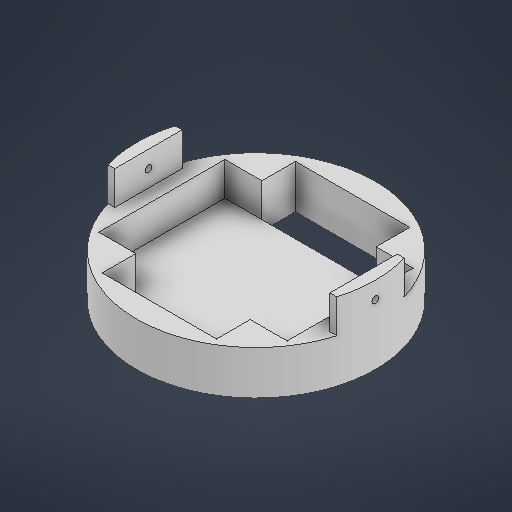
# Autodesk Inventor part: 007-002
Saved by Autodesk Inventor 2026 (Build 300175000, 175)
## iProperties
Created: 2026-04-20
Part Number: 007-002
Material: Ogólny
Document SubType Name: Modeling
Designer: Patryk Lombardo
Density: 1 g/cm^3
Appearance: Domyślna
Author: Patryk Lombardo
Autodesk Inventor part; units mm, degrees
ref_plane "YZ Plane" through (0, 0, 0) normal (1, 0, 0) x (0, 1, 0)
ref_plane "XZ Plane" through (0, 0, 0) normal (0, 1, 0) x (-1, 0, 0)
ref_plane "XY Plane" through (0, 0, 0) normal (0, 0, 1) x (1, 0, 0)
sketch "Szkic1" plane through (0, 0, 0) normal (0, 1, 0) x (-1, 0, 0)
  circle A0 centre (0, 0) radius 35.5
  line L0 (0, 18.75) -> (0, -18.75) construction
  line L1 (-28, 0) -> (28, 0) construction
  line L2 (-28, -18.75) -> (28, -18.75)
  line L3 (-28, 18.75) -> (-28, -18.75)
  line L4 (28, 18.75) -> (28, -18.75)
  line L5 (0, 18.75) -> (28, 18.75)
  line L6 (0, 18.75) -> (-28, 18.75)
  line L7 (0, 18.75) -> (0, 28.75) construction
  line L8 (17, 28.75) -> (-17, 28.75)
  line L9 (17, 28.75) -> (17, 18.75)
  line L10 (-17, 28.75) -> (-17, 18.75)
  line L11 (0, -18.75) -> (0, -28.75) construction
  line L12 (-17, -28.75) -> (17, -28.75)
  line L13 (17, -28.75) -> (17, -18.75)
  line L14 (-17, -28.75) -> (-17, -18.75)
  point P0 (0, 0)
  dimension "d0" = 71
  dimension "d1" = 37.5
  dimension "d2" = 56
  dimension "d3" = 10
  dimension "d4" = 34
  dimension "d5" = 10
  dimension "d6" = 34
  constraints: 30 end point, 7 midpoint, 5 horizontal, 5 vertical, 4 point on line, 3 perpendicular, 2 coincident, 1 centre point, 1 collinear
  measures "d0" diameter of A0
  measures "d1" distance of L0.start L0.end
  measures "d2" distance of L1.start L1.end
  measures "d3" distance of L0.start L7.end
  measures "d4" distance of L8.start L8.end
  measures "d5" distance of L0.end L11.end
  measures "d6" distance of L12.start L12.end
extrude "Wyciągnięcie proste1" add sketch "Szkic1" along normal blind 10
extrude "Wyciągnięcie proste2" add sketch "Szkic1" against normal blind 3 contours A0 | L3 L6 L5 L4 L2
sketch "Szkic2" plane through (0, 10, 0) normal (0, 1, 0) x (1, 0, 0)
  line L0 (32, 0) -> (-32, 0) construction
  circle A0 centre (0, 0) radius 35.5
  line L1 (-32, -10) -> (-32, 10)
  line L2 (32, -10) -> (32, 10)
  line L3 (32, -10) -> (34.0624, -10)
  line L4 (32, 10) -> (34.0624, 10)
  line L5 (-32, -10) -> (-34.0624, -10)
  line L6 (-32, 10) -> (-34.0624, 10)
  point P0 (0, 0)
  dimension "d11" = 64
  dimension "d12" = 71
  dimension "d13" = 20
  dimension "d14" = 20
  constraints: 14 end point, 4 horizontal, 4 point on circle, 3 coincident, 3 midpoint, 2 vertical, 1 centre point, 1 parallel
  measures "d11" distance of L0.start L0.end
  measures "d12" diameter of A0
  measures "d13" distance of L1.start L1.end
  measures "d14" distance of L2.start L2.end
extrude "Wyciągnięcie proste3" add sketch "Szkic2" along normal blind 10 contours A0 L3 L2 L4 | L6 L1 L5 A0
sketch "Szkic3" plane through (-32, 10, 10) normal (1, 0, 0) x (0, 0, -1)
  line L0 (0, 0) -> (10, 0) construction
  line L1 (10, 0) -> (10, 5) construction
  circle A0 centre (10, 5) radius 1
  point P0 (10, -10)
  dimension "d17" = 10
  dimension "d18" = 5
  dimension "d19" = 0
  dimension "d20" = 10
  dimension "d21" = 2
  constraints: 4 end point, 1 centre point, 1 coincident, 1 horizontal, 1 perpendicular
  measures "d17" distance of L0.start L0.end
  measures "d18" distance of L0.end L1.end
  measures "d19" distance from line of point (10, -10) L1
  measures "d20" distance from line of point (10, -10) L0
  measures "d21" diameter of A0
extrude "Wyciągnięcie proste4" cut sketch "Szkic3" along normal through all both and the other way through all
